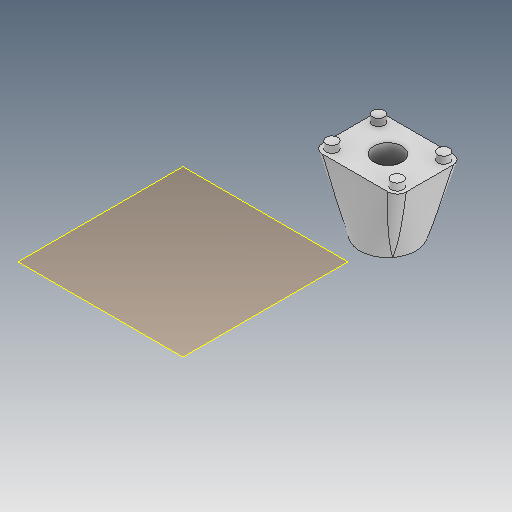
# Autodesk Inventor part: feet
Saved by Autodesk Inventor 2027 (Build 310192060, 192F)
## iProperties
Created: 2026-07-28
Part Number: feet
Material: Generic
Document SubType Name: Modeling
Designer: prest
Density: 1 g/cm^3
Appearance: Default
Author: prest
Autodesk Inventor part; units mm, degrees
ref_plane "YZ Plane" through (0, 0, 0) normal (1, 0, 0) x (0, 1, 0)
ref_plane "XY Plane" through (0, 0, 0) normal (0, 0, 1) x (1, 0, 0)
sketch "Sketch1" plane through (0, 0, 0) normal (0, 1, 0) x (-1, 0, 0)
  circle A0 centre (0, 0) radius 6
  dimension "d1" = 12
  constraints: 1 centre point, 1 coincident
  measures "d1" diameter of A0
ref_plane "Work Plane1" through (0, 15, 0) normal (0, 1, 0) x (-1, 0, 0)
sketch "Sketch2" plane through (0, 15, 0) normal (0, 1, 0) x (-1, 0, 0)
  line L0 (9, 7) -> (-9, 7)
  line L1 (-9, -7) -> (9, -7)
  line L2 (9, -7) -> (9, 7)
  line L3 (-9, 7) -> (-9, -7)
  line L4 (-9, 7) -> (9, -7) construction
  line L5 (-9, -7) -> (9, 7) construction
  point P0 (0, 0)
  point P1 (0, 0)
  dimension "d2" = 14
  dimension "d3" = 18
  constraints: 12 end point, 1 coincident, 1 horizontal, 1 midpoint, 1 parallel, 1 perpendicular, 1 vertical
  measures "d2" distance of L1.end L0.start
  measures "d3" distance of L0.start L0.end
loft "Loft1" add profiles "Sketch1", "Sketch2"
fillet "Fillet1" radius 2 4 edges at (6.8705, 7.5, -5.3387) (6.8705, 7.5, 5.3387) (-6.8705, 7.5, -5.3387) (-6.8705, 7.5, 5.3387)
sketch "Sketch3" plane through (-7.0198, 15, 7) normal (0, 1, 0) x (1, 0, 0)
  circle A0 centre (14.0198, 2) radius 1.25
  dimension "d12" = 2.5
  dimension "d13" = 2
  dimension "d14" = 2
  constraints: 1 centre point, 1 other
  measures "d12" diameter of A0
  measures "d13" horizontal distance of A0.centre point (16.02, 1.949)
  measures "d14" vertical distance of point (14.04, 0) A0.centre
extrude "Extrusion1" add sketch "Sketch3" along normal blind 1.5
mirror "Mirror1" about plane through (0, 0, 0) normal (1, 0, 0) of "Extrusion1"
mirror "Mirror2" about plane through (0, 0, 0) normal (0, 0, 1) of "Extrusion1", "Mirror1"
sketch "Sketch5" plane through (0, 0, 0) normal (0, -1, 0) x (1, 0, 0)
  point P0 (0, 0)
  point P1 (0, 0)
  constraints: 1 coincident
hole "Hole2" at (0, 0, 0) direction (0, 1, 0) diameter 6 end through all countersink diameter 8 countersink angle 90
body "Solid1"
